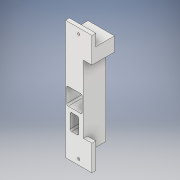
# Autodesk Inventor part: BP005
Saved by Autodesk Inventor 2017 (Build 210142000, 142)
## iProperties
Created: 2018-01-07
Part Number: BP005
Material: ABS Plastic
Document SubType Name: Modeling
Designer: Zach
Density: 1.06 g/cm^3
Appearance: CR White
Author: Zach
Autodesk Inventor part; units mm, degrees
ref_plane "YZ Plane" through (0, 0, 0) normal (1, 0, 0) x (0, 1, 0)
ref_plane "XZ Plane" through (0, 0, 0) normal (0, 1, 0) x (-1, 0, 0)
ref_plane "XY Plane" through (0, 0, 0) normal (0, 0, 1) x (1, 0, 0)
sketch "Sketch1" plane through (0, 0, 0) normal (0, 0, 1) x (1, 0, 0)
  line L0 (0, 0) -> (34, 0)
  line L1 (34, 0) -> (34, 153)
  line L2 (34, 153) -> (0, 153)
  line L3 (0, 153) -> (0, 0)
  circle A0 centre (17, 7) radius 1.5
  circle A1 centre (17, 146) radius 1.5
  point P0 (17, 153)
  point P1 (17, 0)
  dimension "d0" = 34
  dimension "d1" = 153
  dimension "d2" = 3
  dimension "d4" = 7
  dimension "d5" = 3
  dimension "d6" = 7
  constraints: 8 end point, 2 centre point, 2 midpoint, 2 parallel, 2 vertical alignment, 1 horizontal, 1 perpendicular
  measures "d0" distance of L2.end L1.end
  measures "d1" distance of L1.end L0.end
  measures "d2" diameter of A0
  measures "d4" distance from line of L0 A0.centre
  measures "d5" diameter of A1
  measures "d6" distance from line of L2 A1.centre
extrude "Extrusion1" add sketch "Sketch1" along normal blind 5
sketch "Sketch2" plane through (0, 0, 0) normal (0, 0, -1) x (-1, 0, 0)
  line L0 (0, 153) -> (0, 0) projected
  line L1 (0, 138) -> (-34, 138)
  line L2 (-34, 138) -> (-34, 15)
  line L3 (-34, 15) -> (0, 15)
  line L4 (0, 15) -> (0, 138)
  line L5 (-34, 0) -> (-34, 153) projected
  point P0 (0, 76.5)
  dimension "d10" = 123
  constraints: 8 end point, 2 midpoint, 2 parallel, 2 point on line, 1 horizontal, 1 perpendicular
  measures "d10" distance of L2.end L1.end
extrude "Extrusion2" add sketch "Sketch2" along normal blind 5
sketch "Sketch3" plane through (0, 0, 5) normal (0, 0, 1) x (1, 0, 0)
  line L0 (23, 33) -> (34, 33)
  line L1 (34, 33) -> (34, 120)
  line L2 (34, 120) -> (23, 120)
  line L3 (23, 120) -> (23, 33)
  line L4 (34, 0) -> (34, 153) construction
  line L5 (0, 15) -> (34, 15) construction
  line L6 (34, 138) -> (0, 138) construction
  line L7 (28.5, 33) -> (28.5, 15) construction
  line L8 (28.5, 120) -> (28.5, 138) construction
  dimension "d29" = 11
  dimension "d30" = 87
  constraints: 12 end point, 3 point on line, 2 midpoint, 2 parallel, 2 perpendicular, 1 collinear, 1 horizontal, 1 vertical
  measures "d29" distance of L2.end L1.end
  measures "d30" distance of L1.end L0.end
extrude "Extrusion3" cut sketch "Sketch3" against normal through all
sketch "Sketch4" plane through (0, 0, 5) normal (0, 0, 1) x (1, 0, 0)
  line L0 (17, 33) -> (6, 33)
  line L1 (6, 33) -> (6, 54)
  line L2 (6, 54) -> (17, 54)
  line L3 (17, 54) -> (17, 33)
  line L4 (23, 33) -> (23, 120)
  line L5 (0, 153) -> (0, 0)
  line L6 (6, 43.5) -> (0, 43.5)
  line L7 (17, 43.5) -> (23, 43.5)
  dimension "d17" = 11
  dimension "d18" = 21
  constraints: 16 end point, 4 coincident, 3 point on line, 2 midpoint, 2 parallel, 2 perpendicular, 1 collinear, 1 horizontal, 1 horizontal alignment
  measures "d17" distance of L1.end L2.end
  measures "d18" distance of L0.end L1.end
extrude "Extrusion4" cut sketch "Sketch4" against normal through all
fillet "Fillet1" radius 2 4 edges at (6, 54, 0) (17, 54, 0) (17, 33, 0) (6, 33, 0)
sketch "Sketch6" plane through (0, 0, 5) normal (0, 0, 1) x (1, 0, 0)
  line L0 (21.5, 59) -> (1.5, 59)
  line L1 (1.5, 59) -> (1.5, 81)
  line L2 (1.5, 81) -> (21.5, 81)
  line L3 (21.5, 81) -> (21.5, 59)
  line L4 (17, 34) -> (17, 17) construction
  line L5 (8, 54) -> (15, 54) construction
  line L6 (1.5, 70) -> (0, 70) construction
  line L7 (0, 153) -> (0, 0) construction
  line L8 (21.5, 70) -> (23, 70) construction
  line L9 (23, 33) -> (23, 120)
  dimension "d23" = 20
  dimension "d24" = 22
  dimension "d25" = 5
  constraints: 20 end point, 5 coincident, 3 point on line, 2 horizontal, 2 midpoint, 2 parallel, 1 collinear, 1 perpendicular
  measures "d23" distance of L1.end L2.end
  measures "d24" distance of L0.end L1.end
  measures "d25" distance between parallel lines of L5 L0
extrude "Extrusion5" cut sketch "Sketch6" against normal through all
fillet "Fillet2" radius 2 4 edges at (21.5, 81, 0) (1.5, 81, 0) (1.5, 59, 0) (21.5, 59, 0)
sketch "Sketch7" plane through (0, 0, -5) normal (0, 0, -1) x (-1, 0, 0)
  line L0 (-21.5, 61) -> (-21.5, 79) projected
  arc A0 (-19.5, 81) -> (-21.5, 79) centre (-19.5, 79) ccw projected
  line L1 (-19.5, 81) -> (-3.5, 81) projected
  arc A1 (-1.5, 79) -> (-3.5, 81) centre (-3.5, 79) ccw projected
  line L2 (-1.5, 79) -> (-1.5, 61) projected
  arc A2 (-3.5, 59) -> (-1.5, 61) centre (-3.5, 61) ccw projected
  line L3 (-3.5, 59) -> (-19.5, 59) projected
  arc A3 (-21.5, 61) -> (-19.5, 59) centre (-19.5, 61) ccw projected
  line L4 (-17, 35) -> (-17, 52) projected
  arc A4 (-15, 54) -> (-17, 52) centre (-15, 52) ccw projected
  line L5 (-15, 54) -> (-8, 54) projected
  arc A5 (-6, 52) -> (-8, 54) centre (-8, 52) ccw projected
  line L6 (-6, 52) -> (-6, 35) projected
  arc A6 (-8, 33) -> (-6, 35) centre (-8, 35) ccw projected
  line L7 (-8, 33) -> (-15, 33) projected
  arc A7 (-17, 35) -> (-15, 33) centre (-15, 35) ccw projected
  line L8 (-23, 33) -> (-34, 33) projected
  line L9 (-34, 33) -> (-34, 15) projected
  line L10 (-34, 15) -> (0, 15) projected
  line L11 (0, 15) -> (0, 138) projected
  line L12 (0, 138) -> (-34, 138) projected
  line L13 (-34, 138) -> (-34, 120) projected
  line L14 (-34, 120) -> (-23, 120) projected
  line L15 (-23, 120) -> (-23, 33) projected
  point P0 (0, 0)
extrude "Extrusion6" add sketch "Sketch7" along normal blind 19
sketch "Sketch8" plane through (23, 33, 5) normal (0, 1, 0) x (1, 0, 0)
  line L0 (0, 0) -> (0, 29) projected
  line L1 (11, 0) -> (0, 0) projected
  line L2 (11, 29) -> (11, 0) projected
  line L3 (0, 29) -> (11, 29) projected
  line L4 (-23, 5) -> (11, 5) projected
  line L5 (0, 5) -> (11, 5)
  constraints: 2 end point, 2 point on line, 1 perpendicular
extrude "Extrusion7" cut sketch "Sketch8" against normal through all contours L0 L3 L2 L4
body "Solid1"
